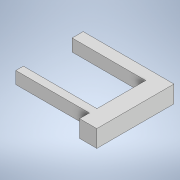
# Autodesk Inventor part: JoystickHållare
Saved by Autodesk Inventor 2021 (Build 250183000, 183)
## iProperties
Created: 2024-03-26
Part Number: JoystickHållare
Material: Generic
Document SubType Name: Modeling
Designer: 21seblin
Density: 1 g/cm^3
Appearance: Default
Author: 21seblin
Autodesk Inventor part; units mm, degrees
ref_plane "YZ Plane" through (0, 0, 0) normal (1, 0, 0) x (0, 1, 0)
ref_plane "XZ Plane" through (0, 0, 0) normal (0, 1, 0) x (-1, 0, 0)
ref_plane "XY Plane" through (0, 0, 0) normal (0, 0, 1) x (1, 0, 0)
sketch "Sketch1" plane through (0, 0, 0) normal (0, 1, 0) x (-1, 0, 0)
  line L0 (-3.5, 15.724) -> (3.5, 15.724)
  line L1 (3.5, 15.724) -> (3.5, -15.724)
  line L2 (3.5, -15.724) -> (-3.5, -15.724)
  line L3 (-3.5, -15.724) -> (-3.5, 15.724)
  line L4 (-3.5, 15.724) -> (3.5, -15.724) construction
  line L5 (3.5, 15.724) -> (-3.5, -15.724) construction
  line L6 (3.5, 15.724) -> (3.5, 11.724)
  point P0 (0, 0)
  dimension "d0" = 7
  dimension "d1" = 4
  constraints: 14 end point, 2 midpoint, 2 parallel, 1 horizontal, 1 perpendicular, 1 point on line
  measures "d0" distance of L1.end L2.end
  measures "d1" distance of L0.end L6.end
extrude "Extrusion1" add sketch "Sketch1" along normal blind 7
sketch "Sketch2" plane through (-3.5, 0, -15.724) normal (-1, 0, 0) x (0, 0, 1)
  line L0 (31.4479, 7) -> (0, 7) projected
  line L1 (31.4479, 7) -> (27.4406, 7)
  line L2 (0, 7) -> (4.5, 7)
  line L3 (4.5, 7) -> (4.5, 2.0159)
  line L4 (4.5, 2.0159) -> (0, 2.0159)
  line L5 (0, 2.0159) -> (0, 7)
  line L6 (27.4406, 7) -> (24.383, 7)
  line L7 (24.383, 7) -> (24.383, 2.0159)
  line L8 (24.383, 2.0159) -> (27.4406, 2.0159)
  line L9 (27.4406, 2.0159) -> (27.4406, 7)
  point P0 (15.724, 0)
  point P1 (4.5, 7)
  dimension "d4" = 4.5
  constraints: 18 end point, 4 parallel, 2 horizontal, 2 perpendicular, 1 point on line
  measures "d4" distance of L3.end L4.end
extrude "Extrusion2" add sketch "Sketch2" along normal blind 30
body "Solid1"
